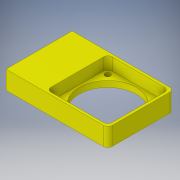
# Autodesk Inventor part: Fan_Bracket
Saved by Autodesk Inventor 2016 (Build 200138000, 138)
## iProperties
Created: 2016-05-21
Part Number: Fan_Bracket
Material: ABS Plastic
Document SubType Name: Modeling
Designer: agmle
Density: 1.06 g/cm^3
Appearance: Smooth - Yellow
Author: agmle
Autodesk Inventor part; units mm, degrees
ref_plane "YZ Plane" through (0, 0, 0) normal (1, 0, 0) x (0, 1, 0)
ref_plane "XZ Plane" through (0, 0, 0) normal (0, 1, 0) x (-1, 0, 0)
ref_plane "XY Plane" through (0, 0, 0) normal (0, 0, 1) x (1, 0, 0)
sketch "Sketch1" plane through (0, 0, 0) normal (0, 1, 0) x (-1, 0, 0)
  line L0 (3.62, 0) -> (84.271, 0)
  line L1 (84.271, 0) -> (84.271, -54.75)
  line L2 (84.271, -54.75) -> (3.62, -54.75)
  line L3 (0, -51.13) -> (0, -3.62)
  circle A0 centre (27.375, -27.375) radius 23.815
  line L4 (0, -27.375) -> (27.375, -27.375) construction
  line L5 (27.375, -27.375) -> (27.375, 0) construction
  arc A1 (0, -51.13) -> (3.62, -54.75) centre (3.62, -51.13) ccw
  arc A2 (3.62, 0) -> (0, -3.62) centre (3.62, -3.62) ccw
  point P0 (0, 0)
  point P1 (0, -54.75)
  dimension "d0" = 54.75
  dimension "d1" = 84.271
  dimension "d2" = 47.63
  dimension "d3" = 3.62
  constraints: 12 end point, 5 point on line, 4 perpendicular, 4 point on circle, 4 tangent, 3 centre point, 2 parallel, 1 equal radius, 1 horizontal, 1 midpoint
  measures "d0" distance of point (0, -54.75) point (0, 0)
  measures "d1" distance of point (0, 0) L0.end
  measures "d2" diameter of A0
  measures "d3" radius of A1
extrude "Extrusion1" add sketch "Sketch1" along normal blind 15.2
sketch "Sketch2" plane through (0, 15.2, 0) normal (0, 1, 0) x (1, 0, 0)
  line L0 (-49.13, 2) -> (-5.62, 2)
  line L1 (-2, 5.62) -> (-2, 49.13)
  line L2 (-5.62, 52.75) -> (-49.13, 52.75)
  line L3 (-52.75, 49.13) -> (-52.75, 5.62)
  circle A0 centre (-27.375, 27.375) radius 23.815 construction
  line L4 (-52.75, 27.375) -> (-2, 27.375) construction
  arc A1 (-52.75, 5.62) -> (-49.13, 2) centre (-49.13, 5.62) ccw
  arc A2 (-49.13, 52.75) -> (-52.75, 49.13) centre (-49.13, 49.13) ccw
  arc A3 (-2, 49.13) -> (-5.62, 52.75) centre (-5.62, 49.13) ccw
  arc A4 (-5.62, 2) -> (-2, 5.62) centre (-5.62, 5.62) ccw
  point P0 (0, 0)
  point P1 (-52.75, 2)
  point P2 (-52.75, 52.75)
  dimension "d6" = 50.75
  dimension "d7" = 3.62
  constraints: 10 end point, 8 point on circle, 8 tangent, 4 centre point, 4 point on line, 3 equal radius, 3 midpoint, 2 parallel, 2 perpendicular, 1 coincident, 1 horizontal
  measures "d6" distance of point (-52.75, 52.75) point (-52.75, 2)
  measures "d7" radius of A1
extrude "Extrusion2" cut sketch "Sketch2" against normal blind 10.2
sketch "Sketch3" plane through (0, 5, 0) normal (0, 1, 0) x (1, 0, 0)
  line L0 (-48.375, 6.375) -> (-6.375, 6.375) construction
  line L1 (-6.375, 6.375) -> (-6.375, 48.375) construction
  line L2 (-6.375, 48.375) -> (-48.375, 48.375) construction
  line L3 (-48.375, 48.375) -> (-48.375, 6.375) construction
  line L4 (-48.375, 27.375) -> (-6.375, 27.375) construction
  circle A0 centre (-27.375, 27.375) radius 23.815 construction
  point P0 (0, 0)
  dimension "d10" = 42
  constraints: 10 end point, 5 coincident, 3 midpoint, 2 parallel, 2 perpendicular, 1 horizontal
  measures "d10" distance of L2.end L0.start
hole "Hole1" at (-48.375, 5, -6.375) at (-48.375, 5, -48.375) at (-6.375, 5, -48.375) at (-6.375, 5, -6.375) direction (0, -1, 0) diameter 4.4958 end through all clearance for "Socket Head Cap Screw" size "M4" standard "Ansi Metric M Profile"
sketch "Sketch4" plane through (-84.271, 0, -54.75) normal (-1, 0, 0) x (0, 0, 1)
  line L0 (0, 0) -> (54.75, 0) construction
  line L1 (54.75, 0) -> (54.75, 15.2) construction
  line L2 (0, 15.2) -> (54.75, 15.2) construction
  line L3 (0, 0) -> (0, 15.2) construction
  line L4 (12.7, 7.6) -> (42.05, 7.6) construction
  line L5 (51.13, 15.2) -> (3.62, 15.2) construction
  line L6 (27.375, 15.2) -> (27.375, 0) construction
  line L7 (51.19, 0) -> (3.56, 0) construction
  point P0 (27.375, 7.6)
  dimension "d18" = 12.7
  dimension "Bracket_Hole_Spacing" = 29.35
  constraints: 4 end point, 4 midpoint, 2 coincident, 1 horizontal
  measures "d18" distance from line of L3 point (12.7, 7.6)
  measures "Bracket_Hole_Spacing" distance of L4.end point (12.7, 7.6)
hole "Hole2" at (-84.271, 7.6, -42.05) at (-84.271, 7.6, -12.7) direction (1, 0, 0) diameter 2.159 depth 25.4 tip angle 118
equation "\"d1\" = Compressor_Center_Offset + 0.5 * d0"
equation "\"d2\" = Fan_ID"
equation "\"d3\" = Fan_Corner_Radius"
equation "\"d7\" = Fan_Corner_Radius"
equation "\"d8\" = Fan_Thickness"
equation "\"d10\" = Fan_Hole_Spacing"
equation "\"Compressor_Center_Offset\" = 56.896"
equation "\"Fan_ID\" = 47.63"
equation "\"Fan_Corner_Radius\" = 3.62"
equation "\"Fan_Thickness\" = 10.2"
equation "\"Fan_Hole_Spacing\" = 42"
body "Solid1"
